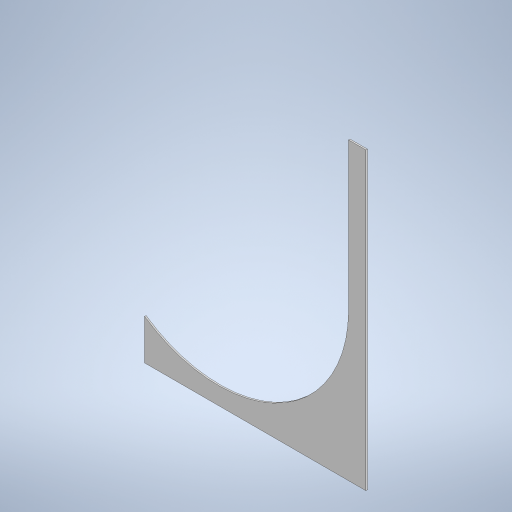
# Autodesk Inventor part: boundaryV1
Saved by Autodesk Inventor 2024.4 (Build 284460000, 460)
## iProperties
Created: 2025-11-05
Part Number: boundaryV1
Material: Generic
Document SubType Name: Modeling
Designer: jonas
Density: 1 g/cm^3
Appearance: Default
Author: jonas
Autodesk Inventor part; units mm, degrees
ref_plane "YZ Plane" through (0, 0, 0) normal (1, 0, 0) x (0, 1, 0)
ref_plane "XZ Plane" through (0, 0, 0) normal (0, 1, 0) x (-1, 0, 0)
ref_plane "XY Plane" through (0, 0, 0) normal (0, 0, 1) x (1, 0, 0)
sketch "Sketch1" plane through (0, 0, 0) normal (0, 1, 0) x (-1, 0, 0)
  line L0 (0, 329.241) -> (0, -329.241) construction
  line L1 (203.5937, 0) -> (-203.5937, 0) construction
  arc A0 (-441.1, 0) -> (250, -363.4133) centre (0, 0) ccw
  line L2 (-441.1, 0) -> (-441.1, 500)
  line L3 (-441.1, 500) -> (-500, 500)
  line L4 (-500, 500) -> (-500, -500)
  line L5 (-500, -500) -> (250, -500)
  line L6 (250, -500) -> (250, -363.4133)
  dimension "d0" = 500
  dimension "d1" = 500
  dimension "d2" = 500
  dimension "d3" = 441.1
  dimension "d4" = 750
  constraints: 14 end point, 4 perpendicular, 2 coincident, 2 midpoint, 2 point on circle, 2 vertical, 1 centre point, 1 horizontal, 1 tangent
  measures "d0" distance between parallel lines of L4 L0
  measures "d1" distance between parallel lines of L3 L1
  measures "d2" distance between parallel lines of L5 L1
  measures "d3" radius of A0
  measures "d4" distance between parallel lines of L4 L6
extrude "Extrusion1" add sketch "Sketch1" along normal blind 5
body "Solid1"
